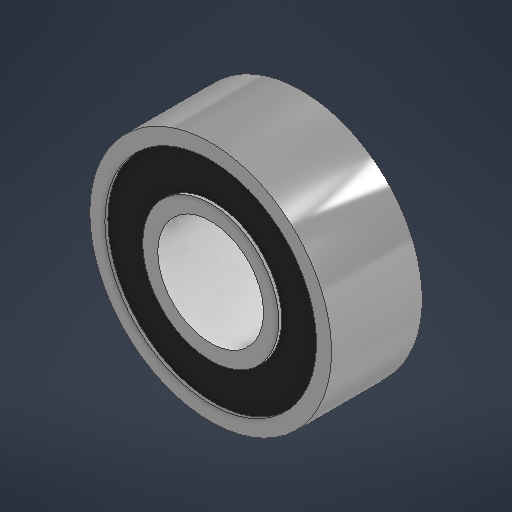
# Autodesk Inventor part: Miniatur Kugellager MR 84 2RS 4x8x3 mm
Saved by Autodesk Inventor 2026.1 (Build 301233020, 233B)
## iProperties
Created: 2025-12-14
Part Number: Miniatur Kugellager MR 84 2RS 4x8x3 mm
Material: Generic
Document SubType Name: Modeling
Designer: Bahaa
Density: 1 g/cm^3
Appearance: Default
Author: Bahaa
Autodesk Inventor part; units mm, degrees
ref_plane "YZ Plane" through (0, 0, 0) normal (1, 0, 0) x (0, 1, 0)
ref_plane "XZ Plane" through (0, 0, 0) normal (0, 1, 0) x (-1, 0, 0)
ref_plane "XY Plane" through (0, 0, 0) normal (0, 0, 1) x (1, 0, 0)
sketch "Sketch1" plane through (0, 0, 0) normal (0, 1, 0) x (-1, 0, 0)
  circle A0 centre (0, 0) radius 4
  circle A1 centre (0, 0) radius 2.25
  circle A2 centre (0, 0) radius 1.75
  circle A3 centre (0, 0) radius 3.5
  dimension "d0" = 8
  dimension "d1" = 4.5
  dimension "d2" = 3.5
  dimension "d3" = 7
  constraints: 4 centre point, 4 coincident
  measures "d0" diameter of A0
  measures "d1" diameter of A1
  measures "d2" diameter of A2
  measures "d3" diameter of A3
extrude "Extrusion1" add sketch "Sketch1" along normal blind 3 contours A0 | A1 | A3
extrude "Extrusion2" cut sketch "Sketch1" against normal blind 0.1 from surface at 3 contours A3
extrude "Extrusion3" cut sketch "Sketch1" along normal blind 0.1 contours A3
body "Solid1"
